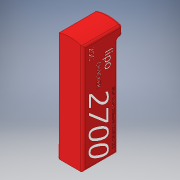
# Autodesk Inventor part: Akku_3S_2700
Saved by Autodesk Inventor 2017 SP1 (Build 210196100, 196)
## iProperties
Part Number: Akku_3S_2700
Material: Generisch
Document SubType Name: Modeling
Designer: Alex
Density: 1 g/cm^3
Appearance: Vorgabe
Author: Alex
Autodesk Inventor part; units mm, degrees
(part 1 of 2)
ref_plane "YZ Plane" through (0, 0, 0) normal (1, 0, 0) x (0, 1, 0)
ref_plane "XZ Plane" through (0, 0, 0) normal (0, 1, 0) x (-1, 0, 0)
ref_plane "XY Plane" through (0, 0, 0) normal (0, 0, 1) x (1, 0, 0)
sketch "Skizze1" plane through (0, 0, 0) normal (0, 1, 0) x (-1, 0, 0)
  line L0 (0, 0) -> (0, -110)
  line L1 (13, 23) -> (13, -138)
  arc A0 (13, 2.5038) -> (0, 0) centre (13, -32.4962) ccw
  line L2 (0, -110) -> (13, -110)
  line L3 (26, 0) -> (26, -110)
  arc A1 (26, 0) -> (13, 2.5038) centre (13, -32.4962) ccw
  line L4 (26, -110) -> (13, -110)
  dimension "d0" = 110
  dimension "d1" = 26
  dimension "d3" = 35
  constraints: 10 end point, 4 point on circle, 2 centre point, 2 point on line, 2 symmetric about line, 2 vertical, 1 perpendicular, 1 other
  measures "d0" distance of L0.start L0.end
  measures "d1" diameter of L0 L1
  measures "d3" radius of A0
extrude "Extrusion1" add sketch "Skizze1" along normal blind 35
sketch "Skizze2" plane through (0, 35, 0) normal (0, 1, 0) x (1, 0, 0)
  arc A0 (-26, 0) -> (0, 0) centre (-13, 32.4962) ccw projected
  arc A1 (-19.9948, -0.0016) -> (0, 0) centre (-10, 33.541) ccw
  line L0 (0, 0) -> (0, 110) projected
  line L1 (-26, 0) -> (-26, 10)
  line L2 (-26, 10) -> (0, 10)
  line L3 (0, 0) -> (0, 10)
  dimension "d6" = 10
  dimension "d7" = 35
  dimension "d8" = 10
  constraints: 6 end point, 2 perpendicular, 2 point on circle, 1 centre point, 1 point on line
  measures "d6" distance from line of L0 A1.centre
  measures "d7" radius of A1
  measures "d8" distance of L1.start L1.end
extrude "Extrusion2" add sketch "Skizze2" along normal blind 5
fillet "Rundung1" radius 2.5 2 edges at (-13, 35, -10) (-13, 40, -10)
fillet "Rundung2" radius 2.5 17 edges at (0, 17.5, -110) (-26, 17.5, -110) (0, 20, 0) (-26, 20, 0) (-13, 40, 2.5038) (0, 39.2678, -9.2678) (0, 37.5, -10) (0, 35.7322, -10.7322) (0, 35, -61.2499) (0, 40, -3.7501) (-26, 37.5, -10) (-26, 35.7322, -10.7322) (-26, 39.2678, -9.2678) (-26, 40, -3.75) (-26, 35, -61.2499) (0, 0, -55) (-26, 0, -55)
sketch "Skizze3" plane through (0, 2.5, -1.739) normal (1, 0, 0) x (0, 0, -1)
  line L0 (47.7852, 29.5) -> (102.261, 29.5) construction
  line L1 (102.261, 29.5) -> (102.261, 25.7703) construction
  line L2 (102.261, 25.7703) -> (47.7852, 25.7703) construction
  line L3 (47.7852, 25.7703) -> (47.7852, 29.5) construction
  line L4 (108.261, -2.5) -> (108.261, 32.5) projected
  line L5 (40.7159, 23.7627) -> (102.0936, 23.7627) construction
  line L6 (102.0936, 23.7627) -> (102.0936, 2.9199) construction
  line L7 (102.0936, 2.9199) -> (40.7159, 2.9199) construction
  line L8 (40.7159, 2.9199) -> (40.7159, 23.7627) construction
  line L9 (108.261, 32.5) -> (10.761, 32.5) projected
  line L10 (2.2367, 27.745) -> (43.751, 27.745) construction
  line L11 (43.751, 27.745) -> (43.751, 1.913) construction
  line L12 (43.751, 1.913) -> (2.2367, 1.913) construction
  line L13 (2.2367, 1.913) -> (2.2367, 27.745) construction
  line L14 (14.308, 19.3885) -> (13.2967, 19.3885)
  line L15 (13.2967, 19.3885) -> (13.2967, 27.745)
  line L16 (13.2967, 27.745) -> (14.308, 27.745)
  line L17 (14.308, 27.745) -> (14.308, 19.3885)
  line L18 (16.8234, 19.3885) -> (15.8121, 19.3885)
  line L19 (15.8121, 19.3885) -> (15.8121, 25.3917)
  line L20 (15.8121, 25.3917) -> (16.8234, 25.3917)
  line L21 (16.8234, 25.3917) -> (16.8234, 19.3885)
  line L22 (16.8947, 26.3901) -> (15.7472, 26.3901)
  line L23 (15.7472, 26.3901) -> (15.7472, 27.4403)
  line L24 (15.7472, 27.4403) -> (16.8947, 27.4403)
  line L25 (16.8947, 27.4403) -> (16.8947, 26.3901)
  spline S0 degree 2 poles (23.3388, 22.5521) (23.3388, 21.0481) (21.9061, 19.2718) (20.8104, 19.2718) knots 0 0 0 1 2 2 2
  spline S1 degree 2 poles (20.8104, 19.2718) (20.3631, 19.2718) (19.6759, 19.4792) (19.3194, 19.6932) knots 0 0 0 1 2 2 2
  line L26 (19.3194, 19.6932) -> (19.3194, 17.1778)
  line L27 (19.3194, 17.1778) -> (18.308, 17.1778)
  line L28 (18.308, 17.1778) -> (18.308, 25.3917)
  line L29 (18.308, 25.3917) -> (19.3194, 25.3917)
  line L30 (19.3194, 25.3917) -> (19.3194, 24.7628)
  spline S2 degree 2 poles (19.3194, 24.7628) (19.6954, 25.1064) (20.6159, 25.5603) (21.154, 25.5603) knots 0 0 0 1 2 2 2
  spline S3 degree 2 poles (21.154, 25.5603) (22.1848, 25.5603) (23.3388, 23.9265) (23.3388, 22.5521) knots 0 0 0 1 2 2 2
  spline S4 degree 2 poles (22.295, 22.4355) (22.295, 23.4662) (21.6403, 24.6008) (20.9077, 24.6008) knots 0 0 0 1 2 2 2
  spline S5 degree 2 poles (20.9077, 24.6008) (20.4798, 24.6008) (19.6759, 24.2183) (19.3194, 23.9201) knots 0 0 0 1 2 2 2
  line L31 (19.3194, 23.9201) -> (19.3194, 20.51)
  spline S6 degree 2 poles (19.3194, 20.51) (19.7148, 20.322) (20.2788, 20.1794) (20.6419, 20.1794) knots 0 0 0 1 2 2 2
  spline S7 degree 2 poles (20.6419, 20.1794) (21.4263, 20.1794) (22.295, 21.3333) (22.295, 22.4355) knots 0 0 0 1 2 2 2
  spline S8 degree 2 poles (29.3226, 22.3901) (29.3226, 20.8731) (27.8639, 19.2199) (26.6451, 19.2199) knots 0 0 0 1 2 2 2
  spline S9 degree 2 poles (26.6451, 19.2199) (25.3939, 19.2199) (23.9612, 20.9249) (23.9612, 22.3901) knots 0 0 0 1 2 2 2
  spline S10 degree 2 poles (23.9612, 22.3901) (23.9612, 23.8941) (25.4393, 25.5603) (26.6451, 25.5603) knots 0 0 0 1 2 2 2
  spline S11 degree 2 poles (26.6451, 25.5603) (27.8639, 25.5603) (29.3226, 23.9006) (29.3226, 22.3901) knots 0 0 0 1 2 2 2
  spline S12 degree 2 poles (28.2788, 22.3901) (28.2788, 23.557) (27.4296, 24.6915) (26.6451, 24.6915) knots 0 0 0 1 2 2 2
  spline S13 degree 2 poles (26.6451, 24.6915) (25.8607, 24.6915) (25.0049, 23.557) (25.0049, 22.3901) knots 0 0 0 1 2 2 2
  spline S14 degree 2 poles (25.0049, 22.3901) (25.0049, 21.2556) (25.8607, 20.0886) (26.6451, 20.0886) knots 0 0 0 1 2 2 2
  spline S15 degree 2 poles (26.6451, 20.0886) (27.4231, 20.0886) (28.2788, 21.2361) (28.2788, 22.3901) knots 0 0 0 1 2 2 2
  spline S16 degree 2 poles (20.7399, 11.1877) (20.351, 11.1877) (19.6929, 11.4502) (19.4531, 11.7128) knots 0 0 0 1 2 2 2
  spline S17 degree 2 poles (19.4531, 11.7128) (19.2132, 11.9721) (18.9506, 12.7501) (18.9506, 13.2557) knots 0 0 0 1 2 2 2
  spline S18 degree 2 poles (18.9506, 13.2557) (18.9506, 13.7582) (19.2067, 14.5037) (19.4498, 14.7792) knots 0 0 0 1 2 2 2
  spline S19 degree 2 poles (19.4498, 14.7792) (19.6897, 15.0483) (20.3445, 15.3303) (20.7497, 15.3303) knots 0 0 0 1 2 2 2
  spline S20 degree 2 poles (20.7497, 15.3303) (20.9506, 15.3303) (21.304, 15.2719) (21.4531, 15.2266) knots 0 0 0 1 2 2 2
  spline S21 degree 2 poles (21.4531, 15.2266) (21.5827, 15.1844) (21.8518, 15.0645) (21.9847, 14.9932) knots 0 0 0 1 2 2 2
  line L32 (21.9847, 14.9932) -> (21.9847, 14.3514)
  line L33 (21.9847, 14.3514) -> (21.9425, 14.3514)
  spline S22 degree 2 poles (21.9425, 14.3514) (21.8712, 14.4162) (21.6508, 14.5977) (21.492, 14.6852) knots 0 0 0 1 2 2 2
  spline S23 degree 2 poles (21.492, 14.6852) (21.3396, 14.7695) (20.9798, 14.8765) (20.7464, 14.8765) knots 0 0 0 1 2 2 2
  spline S24 degree 2 poles (20.7464, 14.8765) (20.4903, 14.8765) (20.0333, 14.6658) (19.8615, 14.4648) knots 0 0 0 1 2 2 2
  spline S25 degree 2 poles (19.8615, 14.4648) (19.6929, 14.2606) (19.5049, 13.6415) (19.5049, 13.2557) knots 0 0 0 1 2 2 2
  spline S26 degree 2 poles (19.5049, 13.2557) (19.5049, 12.8441) (19.7027, 12.2509) (19.8745, 12.0467) knots 0 0 0 1 2 2 2
  spline S27 degree 2 poles (19.8745, 12.0467) (20.043, 11.8489) (20.4936, 11.648) (20.7464, 11.648) knots 0 0 0 1 2 2 2
  spline S28 degree 2 poles (20.7464, 11.648) (20.9766, 11.648) (21.3688, 11.7614) (21.5211, 11.8457) knots 0 0 0 1 2 2 2
  spline S29 degree 2 poles (21.5211, 11.8457) (21.667, 11.93) (21.8842, 12.105) (21.9458, 12.1666) knots 0 0 0 1 2 2 2
  line L34 (21.9458, 12.1666) -> (21.9847, 12.1666)
  line L35 (21.9847, 12.1666) -> (21.9847, 11.5313)
  spline S30 degree 2 poles (21.9847, 11.5313) (21.8518, 11.4697) (21.6184, 11.3562) (21.4531, 11.3044) knots 0 0 0 1 2 2 2
  spline S31 degree 2 poles (21.4531, 11.3044) (21.278, 11.246) (20.9798, 11.1877) (20.7399, 11.1877) knots 0 0 0 1 2 2 2
  line L36 (25.5762, 11.259) -> (24.8858, 11.259)
  line L37 (24.8858, 11.259) -> (23.6216, 12.8506)
  line L38 (23.6216, 12.8506) -> (23.0122, 12.8506)
  line L39 (23.0122, 12.8506) -> (23.0122, 11.259)
  line L40 (23.0122, 11.259) -> (22.4806, 11.259)
  line L41 (22.4806, 11.259) -> (22.4806, 15.259)
  line L42 (22.4806, 15.259) -> (23.5114, 15.259)
  spline S32 degree 2 poles (23.5114, 15.259) (23.855, 15.259) (24.3185, 15.1844) (24.5292, 15.0483) knots 0 0 0 1 2 2 2
  spline S33 degree 2 poles (24.5292, 15.0483) (24.7399, 14.9121) (24.983, 14.4875) (24.983, 14.1731) knots 0 0 0 1 2 2 2
  spline S34 degree 2 poles (24.983, 14.1731) (24.983, 13.7355) (24.5357, 13.1423) (24.1532, 12.9997) knots 0 0 0 1 2 2 2
  line L43 (24.1532, 12.9997) -> (25.5762, 11.259)
  spline S35 degree 2 poles (24.4288, 14.1309) (24.4288, 14.306) (24.3056, 14.575) (24.1759, 14.6625) knots 0 0 0 1 2 2 2
  spline S36 degree 2 poles (24.1759, 14.6625) (24.0625, 14.7371) (23.761, 14.7987) (23.5406, 14.7987) knots 0 0 0 1 2 2 2
  line L44 (23.5406, 14.7987) -> (23.0122, 14.7987)
  line L45 (23.0122, 14.7987) -> (23.0122, 13.2946)
  line L46 (23.0122, 13.2946) -> (23.479, 13.2946)
  spline S37 degree 2 poles (23.479, 13.2946) (23.7091, 13.2946) (24.0754, 13.3757) (24.2018, 13.5021) knots 0 0 0 1 2 2 2
  spline S38 degree 2 poles (24.2018, 13.5021) (24.3185, 13.6123) (24.4288, 13.9235) (24.4288, 14.1309) knots 0 0 0 1 2 2 2
  line L47 (25.4628, 11.259) -> (26.8112, 15.259)
  line L48 (26.8112, 15.259) -> (27.466, 15.259)
  line L49 (27.466, 15.259) -> (28.8145, 11.259)
  line L50 (28.8145, 11.259) -> (28.2537, 11.259)
  line L51 (28.2537, 11.259) -> (27.8907, 12.3773)
  line L52 (27.8907, 12.3773) -> (26.3639, 12.3773)
  line L53 (26.3639, 12.3773) -> (26.0009, 11.259)
  line L54 (26.0009, 11.259) -> (25.4628, 11.259)
  line L55 (27.7448, 12.8311) -> (27.1257, 14.7144)
  line L56 (27.1257, 14.7144) -> (26.5098, 12.8311)
  line L57 (26.5098, 12.8311) -> (27.7448, 12.8311)
  spline S39 degree 2 poles (30.7561, 11.1877) (30.3672, 11.1877) (29.7091, 11.4502) (29.4693, 11.7128) knots 0 0 0 1 2 2 2
  spline S40 degree 2 poles (29.4693, 11.7128) (29.2294, 11.9721) (28.9668, 12.7501) (28.9668, 13.2557) knots 0 0 0 1 2 2 2
  spline S41 degree 2 poles (28.9668, 13.2557) (28.9668, 13.7582) (29.2229, 14.5037) (29.466, 14.7792) knots 0 0 0 1 2 2 2
  spline S42 degree 2 poles (29.466, 14.7792) (29.7059, 15.0483) (30.3607, 15.3303) (30.7659, 15.3303) knots 0 0 0 1 2 2 2
  spline S43 degree 2 poles (30.7659, 15.3303) (30.9668, 15.3303) (31.3202, 15.2719) (31.4693, 15.2266) knots 0 0 0 1 2 2 2
  spline S44 degree 2 poles (31.4693, 15.2266) (31.5989, 15.1844) (31.868, 15.0645) (32.0009, 14.9932) knots 0 0 0 1 2 2 2
  line L58 (32.0009, 14.9932) -> (32.0009, 14.3514)
  line L59 (32.0009, 14.3514) -> (31.9587, 14.3514)
  spline S45 degree 2 poles (31.9587, 14.3514) (31.8874, 14.4162) (31.667, 14.5977) (31.5082, 14.6852) knots 0 0 0 1 2 2 2
  spline S46 degree 2 poles (31.5082, 14.6852) (31.3558, 14.7695) (30.996, 14.8765) (30.7626, 14.8765) knots 0 0 0 1 2 2 2
  spline S47 degree 2 poles (30.7626, 14.8765) (30.5065, 14.8765) (30.0495, 14.6658) (29.8777, 14.4648) knots 0 0 0 1 2 2 2
  spline S48 degree 2 poles (29.8777, 14.4648) (29.7091, 14.2606) (29.5211, 13.6415) (29.5211, 13.2557) knots 0 0 0 1 2 2 2
  spline S49 degree 2 poles (29.5211, 13.2557) (29.5211, 12.8441) (29.7189, 12.2509) (29.8907, 12.0467) knots 0 0 0 1 2 2 2
  spline S50 degree 2 poles (29.8907, 12.0467) (30.0592, 11.8489) (30.5098, 11.648) (30.7626, 11.648) knots 0 0 0 1 2 2 2
  spline S51 degree 2 poles (30.7626, 11.648) (30.9928, 11.648) (31.385, 11.7614) (31.5373, 11.8457) knots 0 0 0 1 2 2 2
  spline S52 degree 2 poles (31.5373, 11.8457) (31.6832, 11.93) (31.9004, 12.105) (31.962, 12.1666) knots 0 0 0 1 2 2 2
  line L60 (31.962, 12.1666) -> (32.0009, 12.1666)
  line L61 (32.0009, 12.1666) -> (32.0009, 11.5313)
  spline S53 degree 2 poles (32.0009, 11.5313) (31.868, 11.4697) (31.6346, 11.3562) (31.4693, 11.3044) knots 0 0 0 1 2 2 2
  spline S54 degree 2 poles (31.4693, 11.3044) (31.2942, 11.246) (30.996, 11.1877) (30.7561, 11.1877) knots 0 0 0 1 2 2 2
  line L62 (35.4142, 11.259) -> (34.7237, 11.259)
  line L63 (34.7237, 11.259) -> (33.2618, 13.1196)
  line L64 (33.2618, 13.1196) -> (33.0284, 12.857)
  line L65 (33.0284, 12.857) -> (33.0284, 11.259)
  line L66 (33.0284, 11.259) -> (32.4968, 11.259)
  line L67 (32.4968, 11.259) -> (32.4968, 15.259)
  line L68 (32.4968, 15.259) -> (33.0284, 15.259)
  line L69 (33.0284, 15.259) -> (33.0284, 13.4211)
  line L70 (33.0284, 13.4211) -> (34.6686, 15.259)
  line L71 (34.6686, 15.259) -> (35.3169, 15.259)
  line L72 (35.3169, 15.259) -> (33.6605, 13.4729)
  line L73 (33.6605, 13.4729) -> (35.4142, 11.259)
  line L74 (35.7318, 11.259) -> (35.7318, 15.259)
  line L75 (35.7318, 15.259) -> (38.2343, 15.259)
  line L76 (38.2343, 15.259) -> (38.2343, 14.7857)
  line L77 (38.2343, 14.7857) -> (36.2634, 14.7857)
  line L78 (36.2634, 14.7857) -> (36.2634, 13.6901)
  line L79 (36.2634, 13.6901) -> (38.1014, 13.6901)
  line L80 (38.1014, 13.6901) -> (38.1014, 13.2168)
  line L81 (38.1014, 13.2168) -> (36.2634, 13.2168)
  line L82 (36.2634, 13.2168) -> (36.2634, 11.7322)
  line L83 (36.2634, 11.7322) -> (38.2343, 11.7322)
  line L84 (38.2343, 11.7322) -> (38.2343, 11.259)
  line L85 (38.2343, 11.259) -> (35.7318, 11.259)
  line L86 (41.9134, 11.259) -> (41.2229, 11.259)
  line L87 (41.2229, 11.259) -> (39.9587, 12.8506)
  line L88 (39.9587, 12.8506) -> (39.3493, 12.8506)
  line L89 (39.3493, 12.8506) -> (39.3493, 11.259)
  line L90 (39.3493, 11.259) -> (38.8177, 11.259)
  line L91 (38.8177, 11.259) -> (38.8177, 15.259)
  line L92 (38.8177, 15.259) -> (39.8485, 15.259)
  spline S55 degree 2 poles (39.8485, 15.259) (40.1921, 15.259) (40.6557, 15.1844) (40.8664, 15.0483) knots 0 0 0 1 2 2 2
  spline S56 degree 2 poles (40.8664, 15.0483) (41.0771, 14.9121) (41.3202, 14.4875) (41.3202, 14.1731) knots 0 0 0 1 2 2 2
  spline S57 degree 2 poles (41.3202, 14.1731) (41.3202, 13.7355) (40.8728, 13.1423) (40.4903, 12.9997) knots 0 0 0 1 2 2 2
  line L93 (40.4903, 12.9997) -> (41.9134, 11.259)
  spline S58 degree 2 poles (40.7659, 14.1309) (40.7659, 14.306) (40.6427, 14.575) (40.513, 14.6625) knots 0 0 0 1 2 2 2
  spline S59 degree 2 poles (40.513, 14.6625) (40.3996, 14.7371) (40.0981, 14.7987) (39.8777, 14.7987) knots 0 0 0 1 2 2 2
  line L94 (39.8777, 14.7987) -> (39.3493, 14.7987)
  line L95 (39.3493, 14.7987) -> (39.3493, 13.2946)
  line L96 (39.3493, 13.2946) -> (39.8161, 13.2946)
  spline S60 degree 2 poles (39.8161, 13.2946) (40.0463, 13.2946) (40.4125, 13.3757) (40.539, 13.5021) knots 0 0 0 1 2 2 2
  spline S61 degree 2 poles (40.539, 13.5021) (40.6557, 13.6123) (40.7659, 13.9235) (40.7659, 14.1309) knots 0 0 0 1 2 2 2
  line L97 (5.6848, 3.4125) -> (2.6014, 3.4125)
  line L98 (2.6014, 3.4125) -> (2.6014, 4.1216)
  spline S62 degree 2 poles (2.6014, 4.1216) (2.9336, 4.4336) (3.5252, 5.013) (3.8088, 5.325) knots 0 0 0 1 2 2 2
  spline S63 degree 2 poles (3.8088, 5.325) (4.3801, 5.953) (4.7975, 6.7067) (4.7975, 7.1078) knots 0 0 0 1 2 2 2
  spline S64 degree 2 poles (4.7975, 7.1078) (4.7975, 7.3185) (4.6678, 7.6345) (4.5503, 7.7358) knots 0 0 0 1 2 2 2
  spline S65 degree 2 poles (4.5503, 7.7358) (4.4328, 7.8371) (4.1249, 7.9384) (3.9385, 7.9384) knots 0 0 0 1 2 2 2
  spline S66 degree 2 poles (3.9385, 7.9384) (3.7602, 7.9384) (3.3955, 7.8493) (3.2294, 7.7804) knots 0 0 0 1 2 2 2
  spline S67 degree 2 poles (3.2294, 7.7804) (3.0876, 7.7237) (2.8242, 7.5616) (2.7432, 7.5049) knots 0 0 0 1 2 2 2
  line L99 (2.7432, 7.5049) -> (2.7067, 7.5049)
  line L100 (2.7067, 7.5049) -> (2.7067, 8.218)
  spline S68 degree 2 poles (2.7067, 8.218) (2.9134, 8.3193) (3.6548, 8.5179) (3.9871, 8.5179) knots 0 0 0 1 2 2 2
  spline S69 degree 2 poles (3.9871, 8.5179) (4.6881, 8.5179) (5.4782, 7.7764) (5.4782, 7.1443) knots 0 0 0 1 2 2 2
  spline S70 degree 2 poles (5.4782, 7.1443) (5.4782, 6.8485) (5.3404, 6.3542) (5.2189, 6.1435) knots 0 0 0 1 2 2 2
  spline S71 degree 2 poles (5.2189, 6.1435) (5.0973, 5.9247) (4.7448, 5.4952) (4.5503, 5.2885) knots 0 0 0 1 2 2 2
  spline S72 degree 2 poles (4.5503, 5.2885) (4.2343, 4.9441) (3.4604, 4.2067) (3.2294, 3.9919) knots 0 0 0 1 2 2 2
  line L101 (3.2294, 3.9919) -> (5.6848, 3.9919)
  line L102 (5.6848, 3.9919) -> (5.6848, 3.4125)
  spline S73 degree 2 poles (9.3842, 5.0008) (9.3842, 4.6402) (9.1532, 4.0243) (8.9425, 3.7974) knots 0 0 0 1 2 2 2
  spline S74 degree 2 poles (8.9425, 3.7974) (8.7318, 3.5705) (8.1038, 3.3072) (7.7148, 3.3072) knots 0 0 0 1 2 2 2
  spline S75 degree 2 poles (7.7148, 3.3072) (7.3582, 3.3072) (6.6613, 3.4652) (6.4061, 3.5908) knots 0 0 0 1 2 2 2
  line L103 (6.4061, 3.5908) -> (6.4061, 4.2999)
  line L104 (6.4061, 4.2999) -> (6.4547, 4.2999)
  spline S76 degree 2 poles (6.4547, 4.2999) (6.5317, 4.2431) (6.8194, 4.0973) (6.9936, 4.0324) knots 0 0 0 1 2 2 2
  spline S77 degree 2 poles (6.9936, 4.0324) (7.1921, 3.9636) (7.5203, 3.8866) (7.727, 3.8866) knots 0 0 0 1 2 2 2
  spline S78 degree 2 poles (7.727, 3.8866) (7.9296, 3.8866) (8.3104, 4.0324) (8.4482, 4.1905) knots 0 0 0 1 2 2 2
  spline S79 degree 2 poles (8.4482, 4.1905) (8.5738, 4.3404) (8.7035, 4.7375) (8.7035, 5.0049) knots 0 0 0 1 2 2 2
  spline S80 degree 2 poles (8.7035, 5.0049) (8.7035, 5.2723) (8.5576, 5.6127) (8.4198, 5.7261) knots 0 0 0 1 2 2 2
  spline S81 degree 2 poles (8.4198, 5.7261) (8.278, 5.8517) (7.8566, 5.9571) (7.6014, 5.9571) knots 0 0 0 1 2 2 2
  spline S82 degree 2 poles (7.6014, 5.9571) (7.3258, 5.9571) (6.7788, 5.872) (6.6127, 5.8355) knots 0 0 0 1 2 2 2
  line L105 (6.6127, 5.8355) -> (6.6127, 8.4125)
  line L106 (6.6127, 8.4125) -> (9.3558, 8.4125)
  line L107 (9.3558, 8.4125) -> (9.3558, 7.825)
  line L108 (9.3558, 7.825) -> (7.257, 7.825)
  line L109 (7.257, 7.825) -> (7.257, 6.4919)
  spline S83 degree 2 poles (7.257, 6.4919) (7.3785, 6.5081) (7.6135, 6.5203) (7.7108, 6.5203) knots 0 0 0 1 2 2 2
  spline S84 degree 2 poles (7.7108, 6.5203) (8.0957, 6.5203) (8.6265, 6.3947) (8.8696, 6.2083) knots 0 0 0 1 2 2 2
  spline S85 degree 2 poles (8.8696, 6.2083) (9.1168, 6.0219) (9.3842, 5.4546) (9.3842, 5.0008) knots 0 0 0 1 2 2 2
  spline S86 degree 2 poles (12.2002, 3.3234) (11.714, 3.3234) (10.8915, 3.6516) (10.5916, 3.9798) knots 0 0 0 1 2 2 2
  spline S87 degree 2 poles (10.5916, 3.9798) (10.2918, 4.3039) (9.9636, 5.2764) (9.9636, 5.9085) knots 0 0 0 1 2 2 2
  spline S88 degree 2 poles (9.9636, 5.9085) (9.9636, 6.5365) (10.2837, 7.4684) (10.5876, 7.8128) knots 0 0 0 1 2 2 2
  spline S89 degree 2 poles (10.5876, 7.8128) (10.8874, 8.1491) (11.7059, 8.5016) (12.2124, 8.5016) knots 0 0 0 1 2 2 2
  spline S90 degree 2 poles (12.2124, 8.5016) (12.4636, 8.5016) (12.9053, 8.4287) (13.0916, 8.372) knots 0 0 0 1 2 2 2
  spline S91 degree 2 poles (13.0916, 8.372) (13.2537, 8.3193) (13.59, 8.1694) (13.7561, 8.0803) knots 0 0 0 1 2 2 2
  line L110 (13.7561, 8.0803) -> (13.7561, 7.278)
  line L111 (13.7561, 7.278) -> (13.7035, 7.278)
  spline S92 degree 2 poles (13.7035, 7.278) (13.6143, 7.359) (13.3388, 7.5859) (13.1403, 7.6953) knots 0 0 0 1 2 2 2
  spline S93 degree 2 poles (13.1403, 7.6953) (12.9498, 7.8007) (12.5001, 7.9344) (12.2083, 7.9344) knots 0 0 0 1 2 2 2
  spline S94 degree 2 poles (12.2083, 7.9344) (11.8882, 7.9344) (11.3169, 7.671) (11.1022, 7.4198) knots 0 0 0 1 2 2 2
  spline S95 degree 2 poles (11.1022, 7.4198) (10.8915, 7.1645) (10.6565, 6.3906) (10.6565, 5.9085) knots 0 0 0 1 2 2 2
  spline S96 degree 2 poles (10.6565, 5.9085) (10.6565, 5.3939) (10.9036, 4.6524) (11.1184, 4.3971) knots 0 0 0 1 2 2 2
  spline S97 degree 2 poles (11.1184, 4.3971) (11.3291, 4.1499) (11.8923, 3.8987) (12.2083, 3.8987) knots 0 0 0 1 2 2 2
  spline S98 degree 2 poles (12.2083, 3.8987) (12.496, 3.8987) (12.9863, 4.0405) (13.1767, 4.1459) knots 0 0 0 1 2 2 2
  spline S99 degree 2 poles (13.1767, 4.1459) (13.3591, 4.2512) (13.6305, 4.47) (13.7075, 4.547) knots 0 0 0 1 2 2 2
  line L112 (13.7075, 4.547) -> (13.7561, 4.547)
  line L113 (13.7561, 4.547) -> (13.7561, 3.7529)
  spline S100 degree 2 poles (13.7561, 3.7529) (13.59, 3.6759) (13.2983, 3.5341) (13.0916, 3.4692) knots 0 0 0 1 2 2 2
  spline S101 degree 2 poles (13.0916, 3.4692) (12.8728, 3.3963) (12.5001, 3.3234) (12.2002, 3.3234) knots 0 0 0 1 2 2 2
  line L114 (54.5085, 3.3413) -> (42.1746, 3.3413)
  line L115 (42.1746, 3.3413) -> (43.1308, 6.1776)
  spline S102 degree 2 poles (43.1308, 6.1776) (44.8975, 7.4256) (48.0417, 9.7432) (49.5976, 10.9912) knots 0 0 0 1 2 2 2
  spline S103 degree 2 poles (49.5976, 10.9912) (52.7419, 13.5034) (55.4323, 16.5179) (55.9833, 18.1225) knots 0 0 0 1 2 2 2
  spline S104 degree 2 poles (55.9833, 18.1225) (56.2751, 18.9653) (56.1778, 20.2295) (55.8537, 20.6346) knots 0 0 0 1 2 2 2
  spline S105 degree 2 poles (55.8537, 20.6346) (55.5295, 21.0398) (54.4274, 21.445) (53.6819, 21.445) knots 0 0 0 1 2 2 2
  spline S106 degree 2 poles (53.6819, 21.445) (52.9688, 21.445) (51.3804, 21.0884) (50.6187, 20.8129) knots 0 0 0 1 2 2 2
  spline S107 degree 2 poles (50.6187, 20.8129) (49.9704, 20.586) (48.7062, 19.9377) (48.301, 19.7108) knots 0 0 0 1 2 2 2
  line L116 (48.301, 19.7108) -> (48.1551, 19.7108)
  line L117 (48.1551, 19.7108) -> (49.1276, 22.5633)
  spline S108 degree 2 poles (49.1276, 22.5633) (50.1, 22.9685) (53.3415, 23.7627) (54.6705, 23.7627) knots 0 0 0 1 2 2 2
  spline S109 degree 2 poles (54.6705, 23.7627) (57.4582, 23.7627) (59.6138, 20.7967) (58.7548, 18.2684) knots 0 0 0 1 2 2 2
  spline S110 degree 2 poles (58.7548, 18.2684) (58.3496, 17.0852) (57.1341, 15.1079) (56.3561, 14.2651) knots 0 0 0 1 2 2 2
  spline S111 degree 2 poles (56.3561, 14.2651) (55.562, 13.3899) (53.5846, 11.6719) (52.5312, 10.8453) knots 0 0 0 1 2 2 2
  spline S112 degree 2 poles (52.5312, 10.8453) (50.797, 9.4677) (46.6965, 6.5179) (45.4809, 5.659) knots 0 0 0 1 2 2 2
  line L118 (45.4809, 5.659) -> (55.3026, 5.659)
  line L119 (55.3026, 5.659) -> (54.5085, 3.3413)
  line L120 (75.5295, 20.3429) -> (61.0887, 3.3413)
  line L121 (61.0887, 3.3413) -> (58.2362, 3.3413)
  line L122 (58.2362, 3.3413) -> (73.3739, 20.9912)
  line L123 (73.3739, 20.9912) -> (63.0498, 20.9912)
  line L124 (63.0498, 20.9912) -> (63.844, 23.3413)
  line L125 (63.844, 23.3413) -> (76.5344, 23.3413)
  line L126 (76.5344, 23.3413) -> (75.5295, 20.3429)
  spline S113 degree 2 poles (88.0417, 13.3413) (86.2103, 7.9604) (81.3642, 2.9199) (78.1065, 2.9199) knots 0 0 0 1 2 2 2
  spline S114 degree 2 poles (78.1065, 2.9199) (74.8002, 2.9199) (73.455, 8.0577) (75.2378, 13.3251) knots 0 0 0 1 2 2 2
  spline S115 degree 2 poles (75.2378, 13.3251) (77.0855, 18.7384) (81.9153, 23.7465) (85.173, 23.7465) knots 0 0 0 1 2 2 2
  spline S116 degree 2 poles (85.173, 23.7465) (88.4793, 23.7465) (89.8083, 18.5601) (88.0417, 13.3413) knots 0 0 0 1 2 2 2
  spline S117 degree 2 poles (82.5312, 7.2473) (83.2605, 8.2359) (84.6057, 11.2829) (85.3188, 13.3413) knots 0 0 0 1 2 2 2
  spline S118 degree 2 poles (85.3188, 13.3413) (86.0158, 15.3996) (86.7289, 18.4304) (86.6641, 19.4515) knots 0 0 0 1 2 2 2
  spline S119 degree 2 poles (86.6641, 19.4515) (86.5992, 20.4726) (85.562, 21.526) (84.4274, 21.526) knots 0 0 0 1 2 2 2
  spline S120 degree 2 poles (84.4274, 21.526) (83.3091, 21.526) (81.5101, 20.4726) (80.7321, 19.4191) knots 0 0 0 1 2 2 2
  spline S121 degree 2 poles (80.7321, 19.4191) (79.9866, 18.398) (78.6252, 15.2862) (77.9607, 13.3251) knots 0 0 0 1 2 2 2
  spline S122 degree 2 poles (77.9607, 13.3251) (77.2475, 11.2181) (76.5506, 8.398) (76.5992, 7.2959) knots 0 0 0 1 2 2 2
  spline S123 degree 2 poles (76.5992, 7.2959) (76.6316, 6.2586) (77.7013, 5.1403) (78.8521, 5.1403) knots 0 0 0 1 2 2 2
  spline S124 degree 2 poles (78.8521, 5.1403) (79.9704, 5.1403) (81.7694, 6.1938) (82.5312, 7.2473) knots 0 0 0 1 2 2 2
  spline S125 degree 2 poles (103.0498, 13.3413) (101.2184, 7.9604) (96.3723, 2.9199) (93.1146, 2.9199) knots 0 0 0 1 2 2 2
  spline S126 degree 2 poles (93.1146, 2.9199) (89.8083, 2.9199) (88.4631, 8.0577) (90.2459, 13.3251) knots 0 0 0 1 2 2 2
  spline S127 degree 2 poles (90.2459, 13.3251) (92.0936, 18.7384) (96.9234, 23.7465) (100.1811, 23.7465) knots 0 0 0 1 2 2 2
  spline S128 degree 2 poles (100.1811, 23.7465) (103.4874, 23.7465) (104.8164, 18.5601) (103.0498, 13.3413) knots 0 0 0 1 2 2 2
  spline S129 degree 2 poles (97.5393, 7.2473) (98.2686, 8.2359) (99.6138, 11.2829) (100.3269, 13.3413) knots 0 0 0 1 2 2 2
  spline S130 degree 2 poles (100.3269, 13.3413) (101.0239, 15.3996) (101.737, 18.4304) (101.6722, 19.4515) knots 0 0 0 1 2 2 2
  spline S131 degree 2 poles (101.6722, 19.4515) (101.6073, 20.4726) (100.5701, 21.526) (99.4355, 21.526) knots 0 0 0 1 2 2 2
  spline S132 degree 2 poles (99.4355, 21.526) (98.3172, 21.526) (96.5182, 20.4726) (95.7402, 19.4191) knots 0 0 0 1 2 2 2
  spline S133 degree 2 poles (95.7402, 19.4191) (94.9947, 18.398) (93.6333, 15.2862) (92.9688, 13.3251) knots 0 0 0 1 2 2 2
  spline S134 degree 2 poles (92.9688, 13.3251) (92.2556, 11.2181) (91.5587, 8.398) (91.6073, 7.2959) knots 0 0 0 1 2 2 2
  spline S135 degree 2 poles (91.6073, 7.2959) (91.6398, 6.2586) (92.7094, 5.1403) (93.8602, 5.1403) knots 0 0 0 1 2 2 2
  spline S136 degree 2 poles (93.8602, 5.1403) (94.9785, 5.1403) (96.7775, 6.1938) (97.5393, 7.2473) knots 0 0 0 1 2 2 2
  spline S137 degree 2 poles (48.6422, 29.1515) (48.551, 29.1515) (48.3707, 29.107) (48.2836, 29.0725) knots 0 0 0 1 2 2 2
  spline S138 degree 2 poles (48.2836, 29.0725) (48.2025, 29.0381) (48.083, 28.9652) (48.0364, 28.9327) knots 0 0 0 1 2 2 2
  line L127 (48.0364, 28.9327) -> (48.0161, 28.9327)
  line L128 (48.0161, 28.9327) -> (48.0161, 29.2873)
  spline S139 degree 2 poles (48.0161, 29.2873) (48.1255, 29.346) (48.5003, 29.4412) (48.6685, 29.4412) knots 0 0 0 1 2 2 2
  spline S140 degree 2 poles (48.6685, 29.4412) (48.8387, 29.4412) (49.0919, 29.3724) (49.1952, 29.2994) knots 0 0 0 1 2 2 2
  spline S141 degree 2 poles (49.1952, 29.2994) (49.3046, 29.2204) (49.4181, 28.9915) (49.4181, 28.8375) knots 0 0 0 1 2 2 2
  spline S142 degree 2 poles (49.4181, 28.8375) (49.4181, 28.6309) (49.1466, 28.3189) (48.9562, 28.2784) knots 0 0 0 1 2 2 2
  line L129 (48.9562, 28.2784) -> (48.9562, 28.2541)
  spline S143 degree 2 poles (48.9562, 28.2541) (49.0352, 28.2378) (49.2155, 28.1649) (49.2925, 28.092) knots 0 0 0 1 2 2 2
  spline S144 degree 2 poles (49.2925, 28.092) (49.3695, 28.0211) (49.4667, 27.7942) (49.4667, 27.6301) knots 0 0 0 1 2 2 2
  spline S145 degree 2 poles (49.4667, 27.6301) (49.4667, 27.4619) (49.3512, 27.1763) (49.2459, 27.0669) knots 0 0 0 1 2 2 2
  spline S146 degree 2 poles (49.2459, 27.0669) (49.1365, 26.9534) (48.8265, 26.8359) (48.63, 26.8359) knots 0 0 0 1 2 2 2
  spline S147 degree 2 poles (48.63, 26.8359) (48.4416, 26.8359) (48.0729, 26.9271) (47.9473, 26.9899) knots 0 0 0 1 2 2 2
  line L130 (47.9473, 26.9899) -> (47.9473, 27.3444)
  line L131 (47.9473, 27.3444) -> (47.9716, 27.3444)
  spline S148 degree 2 poles (47.9716, 27.3444) (48.0769, 27.2674) (48.4335, 27.1256) (48.6097, 27.1256) knots 0 0 0 1 2 2 2
  spline S149 degree 2 poles (48.6097, 27.1256) (48.7131, 27.1256) (48.9197, 27.1904) (48.9886, 27.2654) knots 0 0 0 1 2 2 2
  spline S150 degree 2 poles (48.9886, 27.2654) (49.0555, 27.3404) (49.1264, 27.5186) (49.1264, 27.6544) knots 0 0 0 1 2 2 2
  spline S151 degree 2 poles (49.1264, 27.6544) (49.1264, 27.7901) (49.0473, 27.9664) (48.9764, 28.017) knots 0 0 0 1 2 2 2
  spline S152 degree 2 poles (48.9764, 28.017) (48.9055, 28.0677) (48.7131, 28.1062) (48.5996, 28.1062) knots 0 0 0 1 2 2 2
  line L132 (48.5996, 28.1062) -> (48.4578, 28.1062)
  line L133 (48.4578, 28.1062) -> (48.4578, 28.3837)
  line L134 (48.4578, 28.3837) -> (48.5692, 28.3837)
  spline S153 degree 2 poles (48.5692, 28.3837) (48.7941, 28.3837) (49.0777, 28.5985) (49.0777, 28.8031) knots 0 0 0 1 2 2 2
  spline S154 degree 2 poles (49.0777, 28.8031) (49.0777, 28.8983) (49.0048, 29.034) (48.9461, 29.0746) knots 0 0 0 1 2 2 2
  spline S155 degree 2 poles (48.9461, 29.0746) (48.8832, 29.1171) (48.7293, 29.1515) (48.6422, 29.1515) knots 0 0 0 1 2 2 2
  spline S156 degree 2 poles (50.6114, 26.844) (50.3399, 26.844) (49.959, 26.9575) (49.7909, 27.0385) knots 0 0 0 1 2 2 2
  line L135 (49.7909, 27.0385) -> (49.7909, 27.4558)
  line L136 (49.7909, 27.4558) -> (49.8152, 27.4558)
  spline S157 degree 2 poles (49.8152, 27.4558) (49.9793, 27.3019) (50.3946, 27.1317) (50.5871, 27.1317) knots 0 0 0 1 2 2 2
  spline S158 degree 2 poles (50.5871, 27.1317) (50.8626, 27.1317) (51.1442, 27.3606) (51.1442, 27.549) knots 0 0 0 1 2 2 2
  spline S159 degree 2 poles (51.1442, 27.549) (51.1442, 27.6989) (50.9963, 27.8853) (50.8362, 27.9319) knots 0 0 0 1 2 2 2
  spline S160 degree 2 poles (50.8362, 27.9319) (50.7208, 27.9643) (50.5283, 28.0089) (50.3845, 28.0454) knots 0 0 0 1 2 2 2
  spline S161 degree 2 poles (50.3845, 28.0454) (50.2548, 28.0798) (50.0502, 28.1831) (49.9712, 28.2662) knots 0 0 0 1 2 2 2
  spline S162 degree 2 poles (49.9712, 28.2662) (49.8942, 28.3493) (49.8091, 28.5721) (49.8091, 28.718) knots 0 0 0 1 2 2 2
  spline S163 degree 2 poles (49.8091, 28.718) (49.8091, 29.0219) (50.2832, 29.4331) (50.6499, 29.4331) knots 0 0 0 1 2 2 2
  spline S164 degree 2 poles (50.6499, 29.4331) (50.8606, 29.4331) (51.2333, 29.3501) (51.3934, 29.2711) knots 0 0 0 1 2 2 2
  line L137 (51.3934, 29.2711) -> (51.3934, 28.874)
  line L138 (51.3934, 28.874) -> (51.3691, 28.874)
  spline S165 degree 2 poles (51.3691, 28.874) (51.2495, 28.9834) (50.8768, 29.1455) (50.6721, 29.1455) knots 0 0 0 1 2 2 2
  spline S166 degree 2 poles (50.6721, 29.1455) (50.4412, 29.1455) (50.1555, 28.9287) (50.1555, 28.7524) knots 0 0 0 1 2 2 2
  spline S167 degree 2 poles (50.1555, 28.7524) (50.1555, 28.5944) (50.3237, 28.406) (50.4817, 28.3635) knots 0 0 0 1 2 2 2
  spline S168 degree 2 poles (50.4817, 28.3635) (50.5871, 28.3351) (50.893, 28.2622) (50.9943, 28.2318) knots 0 0 0 1 2 2 2
  spline S169 degree 2 poles (50.9943, 28.2318) (51.2516, 28.1528) (51.4906, 27.8347) (51.4906, 27.6017) knots 0 0 0 1 2 2 2
  spline S170 degree 2 poles (51.4906, 27.6017) (51.4906, 27.4538) (51.3711, 27.1702) (51.2637, 27.0709) knots 0 0 0 1 2 2 2
  spline S171 degree 2 poles (51.2637, 27.0709) (51.1442, 26.9615) (50.8403, 26.844) (50.6114, 26.844) knots 0 0 0 1 2 2 2
  line L139 (53.1742, 26.8886) -> (51.9546, 26.8886)
  line L140 (51.9546, 26.8886) -> (51.9546, 27.1438)
  line L141 (51.9546, 27.1438) -> (52.4084, 27.1438)
  line L142 (52.4084, 27.1438) -> (52.4084, 28.8193)
  line L143 (52.4084, 28.8193) -> (51.9546, 28.8193)
  line L144 (51.9546, 28.8193) -> (51.9546, 29.0482)
  spline S172 degree 2 poles (51.9546, 29.0482) (52.2119, 29.0482) (52.455, 29.1941) (52.4712, 29.3967) knots 0 0 0 1 2 2 2
  line L145 (52.4712, 29.3967) -> (52.7305, 29.3967)
  line L146 (52.7305, 29.3967) -> (52.7305, 27.1438)
  line L147 (52.7305, 27.1438) -> (53.1742, 27.1438)
  line L148 (53.1742, 27.1438) -> (53.1742, 26.8886)
  spline S173 degree 2 poles (55.2852, 28.6349) (55.2852, 28.4729) (55.1697, 28.1811) (55.0664, 28.0798) knots 0 0 0 1 2 2 2
  spline S174 degree 2 poles (55.0664, 28.0798) (54.9367, 27.9522) (54.5862, 27.8205) (54.3188, 27.8205) knots 0 0 0 1 2 2 2
  line L149 (54.3188, 27.8205) -> (54.0372, 27.8205)
  line L150 (54.0372, 27.8205) -> (54.0372, 26.8886)
  line L151 (54.0372, 26.8886) -> (53.705, 26.8886)
  line L152 (53.705, 26.8886) -> (53.705, 29.3886)
  line L153 (53.705, 29.3886) -> (54.333, 29.3886)
  spline S175 degree 2 poles (54.333, 29.3886) (54.5559, 29.3886) (54.8679, 29.3156) (54.9874, 29.2326) knots 0 0 0 1 2 2 2
  spline S176 degree 2 poles (54.9874, 29.2326) (55.1272, 29.1374) (55.2852, 28.8436) (55.2852, 28.6349) knots 0 0 0 1 2 2 2
  spline S177 degree 2 poles (54.9388, 28.6248) (54.9388, 28.7545) (54.8496, 28.9449) (54.7584, 29.0057) knots 0 0 0 1 2 2 2
  spline S178 degree 2 poles (54.7584, 29.0057) (54.6794, 29.0583) (54.4687, 29.1009) (54.3127, 29.1009) knots 0 0 0 1 2 2 2
  line L154 (54.3127, 29.1009) -> (54.0372, 29.1009)
  line L155 (54.0372, 29.1009) -> (54.0372, 28.1041)
  line L156 (54.0372, 28.1041) -> (54.2641, 28.1041)
  spline S179 degree 2 poles (54.2641, 28.1041) (54.4667, 28.1041) (54.7159, 28.169) (54.7969, 28.2541) knots 0 0 0 1 2 2 2
  spline S180 degree 2 poles (54.7969, 28.2541) (54.8719, 28.329) (54.9388, 28.5053) (54.9388, 28.6248) knots 0 0 0 1 2 2 2
  line L157 (58.0202, 26.8886) -> (56.8006, 26.8886)
  line L158 (56.8006, 26.8886) -> (56.8006, 27.1438)
  line L159 (56.8006, 27.1438) -> (57.2544, 27.1438)
  line L160 (57.2544, 27.1438) -> (57.2544, 28.8193)
  line L161 (57.2544, 28.8193) -> (56.8006, 28.8193)
  line L162 (56.8006, 28.8193) -> (56.8006, 29.0482)
  spline S181 degree 2 poles (56.8006, 29.0482) (57.0579, 29.0482) (57.301, 29.1941) (57.3172, 29.3967) knots 0 0 0 1 2 2 2
  line L163 (57.3172, 29.3967) -> (57.5765, 29.3967)
  line L164 (57.5765, 29.3967) -> (57.5765, 27.1438)
  line L165 (57.5765, 27.1438) -> (58.0202, 27.1438)
  line L166 (58.0202, 27.1438) -> (58.0202, 26.8886)
  line L167 (59.8962, 26.8886) -> (58.6766, 26.8886)
  line L168 (58.6766, 26.8886) -> (58.6766, 27.1438)
  line L169 (58.6766, 27.1438) -> (59.1304, 27.1438)
  line L170 (59.1304, 27.1438) -> (59.1304, 28.8193)
  line L171 (59.1304, 28.8193) -> (58.6766, 28.8193)
  line L172 (58.6766, 28.8193) -> (58.6766, 29.0482)
  spline S182 degree 2 poles (58.6766, 29.0482) (58.9339, 29.0482) (59.177, 29.1941) (59.1932, 29.3967) knots 0 0 0 1 2 2 2
  line L173 (59.1932, 29.3967) -> (59.4525, 29.3967)
  line L174 (59.4525, 29.3967) -> (59.4525, 27.1438)
  line L175 (59.4525, 27.1438) -> (59.8962, 27.1438)
  line L176 (59.8962, 27.1438) -> (59.8962, 26.8886)
  line L177 (60.893, 26.8886) -> (60.4918, 26.8886)
  line L178 (60.4918, 26.8886) -> (60.4918, 27.3667)
  line L179 (60.4918, 27.3667) -> (60.893, 27.3667)
  line L180 (60.893, 27.3667) -> (60.893, 26.8886)
  line L181 (62.8136, 26.8886) -> (61.5939, 26.8886)
  line L182 (61.5939, 26.8886) -> (61.5939, 27.1438)
  line L183 (61.5939, 27.1438) -> (62.0478, 27.1438)
  line L184 (62.0478, 27.1438) -> (62.0478, 28.8193)
  line L185 (62.0478, 28.8193) -> (61.5939, 28.8193)
  line L186 (61.5939, 28.8193) -> (61.5939, 29.0482)
  spline S183 degree 2 poles (61.5939, 29.0482) (61.8512, 29.0482) (62.0943, 29.1941) (62.1106, 29.3967) knots 0 0 0 1 2 2 2
  line L187 (62.1106, 29.3967) -> (62.3699, 29.3967)
  line L188 (62.3699, 29.3967) -> (62.3699, 27.1438)
  line L189 (62.3699, 27.1438) -> (62.8136, 27.1438)
  line L190 (62.8136, 27.1438) -> (62.8136, 26.8886)
  line L191 (65.1576, 29.3886) -> (64.2965, 26.8886)
  line L192 (64.2965, 26.8886) -> (63.9379, 26.8886)
  line L193 (63.9379, 26.8886) -> (63.0769, 29.3886)
  line L194 (63.0769, 29.3886) -> (63.4335, 29.3886)
  line L195 (63.4335, 29.3886) -> (64.1264, 27.312)
  line L196 (64.1264, 27.312) -> (64.8192, 29.3886)
  line L197 (64.8192, 29.3886) -> (65.1576, 29.3886)
  line L198 (67.9412, 26.8886) -> (66.3995, 26.8886)
  line L199 (66.3995, 26.8886) -> (66.3995, 27.2431)
  spline S184 degree 2 poles (66.3995, 27.2431) (66.5656, 27.3991) (66.8614, 27.6888) (67.0032, 27.8448) knots 0 0 0 1 2 2 2
  spline S185 degree 2 poles (67.0032, 27.8448) (67.2888, 28.1588) (67.4975, 28.5357) (67.4975, 28.7362) knots 0 0 0 1 2 2 2
  spline S186 degree 2 poles (67.4975, 28.7362) (67.4975, 28.8416) (67.4327, 28.9996) (67.3739, 29.0502) knots 0 0 0 1 2 2 2
  spline S187 degree 2 poles (67.3739, 29.0502) (67.3152, 29.1009) (67.1612, 29.1515) (67.068, 29.1515) knots 0 0 0 1 2 2 2
  spline S188 degree 2 poles (67.068, 29.1515) (66.9789, 29.1515) (66.7965, 29.107) (66.7135, 29.0725) knots 0 0 0 1 2 2 2
  spline S189 degree 2 poles (66.7135, 29.0725) (66.6426, 29.0442) (66.5109, 28.9631) (66.4704, 28.9348) knots 0 0 0 1 2 2 2
  line L200 (66.4704, 28.9348) -> (66.4521, 28.9348)
  line L201 (66.4521, 28.9348) -> (66.4521, 29.2913)
  spline S190 degree 2 poles (66.4521, 29.2913) (66.5555, 29.342) (66.9262, 29.4412) (67.0923, 29.4412) knots 0 0 0 1 2 2 2
  spline S191 degree 2 poles (67.0923, 29.4412) (67.4428, 29.4412) (67.8379, 29.0705) (67.8379, 28.7545) knots 0 0 0 1 2 2 2
  spline S192 degree 2 poles (67.8379, 28.7545) (67.8379, 28.6066) (67.769, 28.3594) (67.7082, 28.2541) knots 0 0 0 1 2 2 2
  spline S193 degree 2 poles (67.7082, 28.2541) (67.6474, 28.1447) (67.4712, 27.9299) (67.3739, 27.8266) knots 0 0 0 1 2 2 2
  spline S194 degree 2 poles (67.3739, 27.8266) (67.2159, 27.6544) (66.829, 27.2857) (66.7135, 27.1783) knots 0 0 0 1 2 2 2
  line L202 (66.7135, 27.1783) -> (67.9412, 27.1783)
  line L203 (67.9412, 27.1783) -> (67.9412, 26.8886)
  line L204 (69.8456, 29.0138) -> (68.7637, 26.8886)
  line L205 (68.7637, 26.8886) -> (68.4072, 26.8886)
  line L206 (68.4072, 26.8886) -> (69.5498, 29.0948)
  line L207 (69.5498, 29.0948) -> (68.2593, 29.0948)
  line L208 (68.2593, 29.0948) -> (68.2593, 29.3886)
  line L209 (68.2593, 29.3886) -> (69.8456, 29.3886)
  line L210 (69.8456, 29.3886) -> (69.8456, 29.0138)
  spline S195 degree 2 poles (71.7074, 28.1386) (71.7074, 27.466) (71.3164, 26.8359) (70.9092, 26.8359) knots 0 0 0 1 2 2 2
  spline S196 degree 2 poles (70.9092, 26.8359) (70.4959, 26.8359) (70.1089, 27.4781) (70.1089, 28.1365) knots 0 0 0 1 2 2 2
  spline S197 degree 2 poles (70.1089, 28.1365) (70.1089, 28.8132) (70.4999, 29.4392) (70.9092, 29.4392) knots 0 0 0 1 2 2 2
  spline S198 degree 2 poles (70.9092, 29.4392) (71.3204, 29.4392) (71.7074, 28.7909) (71.7074, 28.1386) knots 0 0 0 1 2 2 2
  spline S199 degree 2 poles (71.2779, 27.3768) (71.3265, 27.5004) (71.367, 27.8813) (71.367, 28.1386) knots 0 0 0 1 2 2 2
  spline S200 degree 2 poles (71.367, 28.1386) (71.367, 28.3959) (71.3265, 28.7747) (71.2759, 28.9024) knots 0 0 0 1 2 2 2
  spline S201 degree 2 poles (71.2759, 28.9024) (71.2252, 29.03) (71.049, 29.1617) (70.9092, 29.1617) knots 0 0 0 1 2 2 2
  spline S202 degree 2 poles (70.9092, 29.1617) (70.7694, 29.1617) (70.5891, 29.03) (70.5364, 28.8983) knots 0 0 0 1 2 2 2
  spline S203 degree 2 poles (70.5364, 28.8983) (70.4858, 28.7707) (70.4493, 28.3817) (70.4493, 28.1365) knots 0 0 0 1 2 2 2
  spline S204 degree 2 poles (70.4493, 28.1365) (70.4493, 27.8732) (70.4817, 27.5207) (70.5344, 27.3829) knots 0 0 0 1 2 2 2
  spline S205 degree 2 poles (70.5344, 27.3829) (70.583, 27.2532) (70.7633, 27.1135) (70.9092, 27.1135) knots 0 0 0 1 2 2 2
  spline S206 degree 2 poles (70.9092, 27.1135) (71.0469, 27.1135) (71.2273, 27.2451) (71.2779, 27.3768) knots 0 0 0 1 2 2 2
  spline S207 degree 2 poles (73.5834, 28.1386) (73.5834, 27.466) (73.1924, 26.8359) (72.7852, 26.8359) knots 0 0 0 1 2 2 2
  spline S208 degree 2 poles (72.7852, 26.8359) (72.3719, 26.8359) (71.9849, 27.4781) (71.9849, 28.1365) knots 0 0 0 1 2 2 2
  spline S209 degree 2 poles (71.9849, 28.1365) (71.9849, 28.8132) (72.376, 29.4392) (72.7852, 29.4392) knots 0 0 0 1 2 2 2
  spline S210 degree 2 poles (72.7852, 29.4392) (73.1965, 29.4392) (73.5834, 28.7909) (73.5834, 28.1386) knots 0 0 0 1 2 2 2
  spline S211 degree 2 poles (73.1539, 27.3768) (73.2025, 27.5004) (73.2431, 27.8813) (73.2431, 28.1386) knots 0 0 0 1 2 2 2
  spline S212 degree 2 poles (73.2431, 28.1386) (73.2431, 28.3959) (73.2025, 28.7747) (73.1519, 28.9024) knots 0 0 0 1 2 2 2
  spline S213 degree 2 poles (73.1519, 28.9024) (73.1012, 29.03) (72.925, 29.1617) (72.7852, 29.1617) knots 0 0 0 1 2 2 2
  spline S214 degree 2 poles (72.7852, 29.1617) (72.6454, 29.1617) (72.4651, 29.03) (72.4124, 28.8983) knots 0 0 0 1 2 2 2
  spline S215 degree 2 poles (72.4124, 28.8983) (72.3618, 28.7707) (72.3253, 28.3817) (72.3253, 28.1365) knots 0 0 0 1 2 2 2
  spline S216 degree 2 poles (72.3253, 28.1365) (72.3253, 27.8732) (72.3577, 27.5207) (72.4104, 27.3829) knots 0 0 0 1 2 2 2
  spline S217 degree 2 poles (72.4104, 27.3829) (72.459, 27.2532) (72.6393, 27.1135) (72.7852, 27.1135) knots 0 0 0 1 2 2 2
  spline S218 degree 2 poles (72.7852, 27.1135) (72.923, 27.1135) (73.1033, 27.2451) (73.1539, 27.3768) knots 0 0 0 1 2 2 2
  line L211 (76.0773, 26.8886) -> (76.0773, 27.9745)
  spline S219 degree 2 poles (76.0773, 27.9745) (76.0773, 28.1041) (76.0571, 28.325) (76.0247, 28.3857) knots 0 0 0 1 2 2 2
  spline S220 degree 2 poles (76.0247, 28.3857) (75.9922, 28.4526) (75.8687, 28.5174) (75.7613, 28.5174) knots 0 0 0 1 2 2 2
  spline S221 degree 2 poles (75.7613, 28.5174) (75.664, 28.5174) (75.4412, 28.3979) (75.3237, 28.2844) knots 0 0 0 1 2 2 2
  spline S222 degree 2 poles (75.3237, 28.2844) (75.3257, 28.2561) (75.3298, 28.1771) (75.3298, 28.1244) knots 0 0 0 1 2 2 2
  line L212 (75.3298, 28.1244) -> (75.3298, 26.8886)
  line L213 (75.3298, 26.8886) -> (75.0137, 26.8886)
  line L214 (75.0137, 26.8886) -> (75.0137, 27.9745)
  spline S223 degree 2 poles (75.0137, 27.9745) (75.0137, 28.1041) (74.9935, 28.325) (74.961, 28.3857) knots 0 0 0 1 2 2 2
  spline S224 degree 2 poles (74.961, 28.3857) (74.9286, 28.4526) (74.805, 28.5174) (74.6977, 28.5174) knots 0 0 0 1 2 2 2
  spline S225 degree 2 poles (74.6977, 28.5174) (74.5964, 28.5174) (74.3715, 28.3898) (74.2661, 28.2905) knots 0 0 0 1 2 2 2
  line L215 (74.2661, 28.2905) -> (74.2661, 26.8886)
  line L216 (74.2661, 26.8886) -> (73.9501, 26.8886)
  line L217 (73.9501, 26.8886) -> (73.9501, 28.7646)
  line L218 (73.9501, 28.7646) -> (74.2661, 28.7646)
  line L219 (74.2661, 28.7646) -> (74.2661, 28.5579)
  spline S226 degree 2 poles (74.2661, 28.5579) (74.3897, 28.6815) (74.6328, 28.8173) (74.7787, 28.8173) knots 0 0 0 1 2 2 2
  spline S227 degree 2 poles (74.7787, 28.8173) (74.9448, 28.8173) (75.2021, 28.6653) (75.269, 28.4931) knots 0 0 0 1 2 2 2
  spline S228 degree 2 poles (75.269, 28.4931) (75.4128, 28.6532) (75.6843, 28.8173) (75.8423, 28.8173) knots 0 0 0 1 2 2 2
  spline S229 degree 2 poles (75.8423, 28.8173) (75.9639, 28.8173) (76.1624, 28.7423) (76.2354, 28.6572) knots 0 0 0 1 2 2 2
  spline S230 degree 2 poles (76.2354, 28.6572) (76.3103, 28.5721) (76.3934, 28.3169) (76.3934, 28.1244) knots 0 0 0 1 2 2 2
  line L220 (76.3934, 28.1244) -> (76.3934, 26.8886)
  line L221 (76.3934, 26.8886) -> (76.0773, 26.8886)
  line L222 (76.5919, 26.8886) -> (77.4347, 29.3886)
  line L223 (77.4347, 29.3886) -> (77.8439, 29.3886)
  line L224 (77.8439, 29.3886) -> (78.6867, 26.8886)
  line L225 (78.6867, 26.8886) -> (78.3362, 26.8886)
  line L226 (78.3362, 26.8886) -> (78.1093, 27.5875)
  line L227 (78.1093, 27.5875) -> (77.1551, 27.5875)
  line L228 (77.1551, 27.5875) -> (76.9282, 26.8886)
  line L229 (76.9282, 26.8886) -> (76.5919, 26.8886)
  line L230 (78.0182, 27.8712) -> (77.6312, 29.0482)
  line L231 (77.6312, 29.0482) -> (77.2463, 27.8712)
  line L232 (77.2463, 27.8712) -> (78.0182, 27.8712)
  line L233 (80.3723, 26.8886) -> (80.0563, 26.8886)
  line L234 (80.0563, 26.8886) -> (80.0563, 27.9583)
  spline S231 degree 2 poles (80.0563, 27.9583) (80.0563, 28.0879) (80.032, 28.3108) (79.9955, 28.3776) knots 0 0 0 1 2 2 2
  spline S232 degree 2 poles (79.9955, 28.3776) (79.957, 28.4485) (79.8192, 28.5174) (79.7017, 28.5174) knots 0 0 0 1 2 2 2
  spline S233 degree 2 poles (79.7017, 28.5174) (79.5842, 28.5174) (79.335, 28.3918) (79.2155, 28.2905) knots 0 0 0 1 2 2 2
  line L235 (79.2155, 28.2905) -> (79.2155, 26.8886)
  line L236 (79.2155, 26.8886) -> (78.8995, 26.8886)
  line L237 (78.8995, 26.8886) -> (78.8995, 29.5)
  line L238 (78.8995, 29.5) -> (79.2155, 29.5)
  line L239 (79.2155, 29.5) -> (79.2155, 28.5559)
  spline S234 degree 2 poles (79.2155, 28.5559) (79.3573, 28.6835) (79.6308, 28.8173) (79.7848, 28.8173) knots 0 0 0 1 2 2 2
  spline S235 degree 2 poles (79.7848, 28.8173) (80.0603, 28.8173) (80.3723, 28.4526) (80.3723, 28.1062) knots 0 0 0 1 2 2 2
  line L240 (80.3723, 28.1062) -> (80.3723, 26.8886)
  line L241 (83.3849, 26.8886) -> (81.8431, 26.8886)
  line L242 (81.8431, 26.8886) -> (81.8431, 27.2431)
  spline S236 degree 2 poles (81.8431, 27.2431) (82.0093, 27.3991) (82.305, 27.6888) (82.4469, 27.8448) knots 0 0 0 1 2 2 2
  spline S237 degree 2 poles (82.4469, 27.8448) (82.7325, 28.1588) (82.9412, 28.5357) (82.9412, 28.7362) knots 0 0 0 1 2 2 2
  spline S238 degree 2 poles (82.9412, 28.7362) (82.9412, 28.8416) (82.8764, 28.9996) (82.8176, 29.0502) knots 0 0 0 1 2 2 2
  spline S239 degree 2 poles (82.8176, 29.0502) (82.7589, 29.1009) (82.6049, 29.1515) (82.5117, 29.1515) knots 0 0 0 1 2 2 2
  spline S240 degree 2 poles (82.5117, 29.1515) (82.4226, 29.1515) (82.2402, 29.107) (82.1572, 29.0725) knots 0 0 0 1 2 2 2
  spline S241 degree 2 poles (82.1572, 29.0725) (82.0862, 29.0442) (81.9546, 28.9631) (81.914, 28.9348) knots 0 0 0 1 2 2 2
  line L243 (81.914, 28.9348) -> (81.8958, 28.9348)
  line L244 (81.8958, 28.9348) -> (81.8958, 29.2913)
  spline S242 degree 2 poles (81.8958, 29.2913) (81.9991, 29.342) (82.3699, 29.4412) (82.536, 29.4412) knots 0 0 0 1 2 2 2
  spline S243 degree 2 poles (82.536, 29.4412) (82.8865, 29.4412) (83.2815, 29.0705) (83.2815, 28.7545) knots 0 0 0 1 2 2 2
  spline S244 degree 2 poles (83.2815, 28.7545) (83.2815, 28.6066) (83.2127, 28.3594) (83.1519, 28.2541) knots 0 0 0 1 2 2 2
  spline S245 degree 2 poles (83.1519, 28.2541) (83.0911, 28.1447) (82.9149, 27.9299) (82.8176, 27.8266) knots 0 0 0 1 2 2 2
  spline S246 degree 2 poles (82.8176, 27.8266) (82.6596, 27.6544) (82.2726, 27.2857) (82.1572, 27.1783) knots 0 0 0 1 2 2 2
  line L245 (82.1572, 27.1783) -> (83.3849, 27.1783)
  line L246 (83.3849, 27.1783) -> (83.3849, 26.8886)
  spline S247 degree 2 poles (83.6503, 28.5762) (83.6503, 28.7686) (83.7759, 29.0887) (83.8853, 29.2042) knots 0 0 0 1 2 2 2
  spline S248 degree 2 poles (83.8853, 29.2042) (83.9886, 29.3156) (84.2905, 29.4392) (84.4444, 29.4392) knots 0 0 0 1 2 2 2
  spline S249 degree 2 poles (84.4444, 29.4392) (84.6166, 29.4392) (84.8962, 29.3237) (84.9995, 29.2143) knots 0 0 0 1 2 2 2
  spline S250 degree 2 poles (84.9995, 29.2143) (85.1292, 29.0766) (85.271, 28.6309) (85.271, 28.2885) knots 0 0 0 1 2 2 2
  spline S251 degree 2 poles (85.271, 28.2885) (85.271, 27.9785) (85.1312, 27.4234) (84.9955, 27.2391) knots 0 0 0 1 2 2 2
  spline S252 degree 2 poles (84.9955, 27.2391) (84.8516, 27.0446) (84.4465, 26.84) (84.1507, 26.84) knots 0 0 0 1 2 2 2
  spline S253 degree 2 poles (84.1507, 26.84) (84.0838, 26.84) (83.9319, 26.8541) (83.867, 26.8744) knots 0 0 0 1 2 2 2
  line L247 (83.867, 26.8744) -> (83.867, 27.1965)
  line L248 (83.867, 27.1965) -> (83.8832, 27.1965)
  spline S254 degree 2 poles (83.8832, 27.1965) (83.9258, 27.1722) (84.1041, 27.1297) (84.1952, 27.1297) knots 0 0 0 1 2 2 2
  spline S255 degree 2 poles (84.1952, 27.1297) (84.5234, 27.1297) (84.8982, 27.5632) (84.9246, 27.9643) knots 0 0 0 1 2 2 2
  spline S256 degree 2 poles (84.9246, 27.9643) (84.7909, 27.8732) (84.5478, 27.7901) (84.4039, 27.7901) knots 0 0 0 1 2 2 2
  spline S257 degree 2 poles (84.4039, 27.7901) (84.2661, 27.7901) (84.0372, 27.8509) (83.9217, 27.938) knots 0 0 0 1 2 2 2
  spline S258 degree 2 poles (83.9217, 27.938) (83.788, 28.0413) (83.6503, 28.3553) (83.6503, 28.5762) knots 0 0 0 1 2 2 2
  spline S259 degree 2 poles (84.9327, 28.3635) (84.9327, 28.6167) (84.8395, 28.9368) (84.7564, 29.0239) knots 0 0 0 1 2 2 2
  spline S260 degree 2 poles (84.7564, 29.0239) (84.6835, 29.1049) (84.5315, 29.1657) (84.4424, 29.1657) knots 0 0 0 1 2 2 2
  spline S261 degree 2 poles (84.4424, 29.1657) (84.2358, 29.1657) (83.9906, 28.8699) (83.9906, 28.5904) knots 0 0 0 1 2 2 2
  spline S262 degree 2 poles (83.9906, 28.5904) (83.9906, 28.4323) (84.0717, 28.2277) (84.1608, 28.1548) knots 0 0 0 1 2 2 2
  spline S263 degree 2 poles (84.1608, 28.1548) (84.2256, 28.1021) (84.3857, 28.0677) (84.4789, 28.0677) knots 0 0 0 1 2 2 2
  spline S264 degree 2 poles (84.4789, 28.0677) (84.5862, 28.0677) (84.8334, 28.1426) (84.9266, 28.2054) knots 0 0 0 1 2 2 2
  spline S265 degree 2 poles (84.9266, 28.2054) (84.9286, 28.2297) (84.9327, 28.3128) (84.9327, 28.3635) knots 0 0 0 1 2 2 2
  line L249 (86.132, 26.8886) -> (85.7309, 26.8886)
  line L250 (85.7309, 26.8886) -> (85.7309, 27.3667)
  line L251 (85.7309, 27.3667) -> (86.132, 27.3667)
  line L252 (86.132, 27.3667) -> (86.132, 26.8886)
  spline S266 degree 2 poles (86.5676, 28.5762) (86.5676, 28.7686) (86.6932, 29.0887) (86.8026, 29.2042) knots 0 0 0 1 2 2 2
  spline S267 degree 2 poles (86.8026, 29.2042) (86.9059, 29.3156) (87.2078, 29.4392) (87.3618, 29.4392) knots 0 0 0 1 2 2 2
  spline S268 degree 2 poles (87.3618, 29.4392) (87.534, 29.4392) (87.8136, 29.3237) (87.9169, 29.2143) knots 0 0 0 1 2 2 2
  spline S269 degree 2 poles (87.9169, 29.2143) (88.0465, 29.0766) (88.1884, 28.6309) (88.1884, 28.2885) knots 0 0 0 1 2 2 2
  spline S270 degree 2 poles (88.1884, 28.2885) (88.1884, 27.9785) (88.0486, 27.4234) (87.9128, 27.2391) knots 0 0 0 1 2 2 2
  spline S271 degree 2 poles (87.9128, 27.2391) (87.769, 27.0446) (87.3638, 26.84) (87.068, 26.84) knots 0 0 0 1 2 2 2
  spline S272 degree 2 poles (87.068, 26.84) (87.0012, 26.84) (86.8492, 26.8541) (86.7844, 26.8744) knots 0 0 0 1 2 2 2
  line L253 (86.7844, 26.8744) -> (86.7844, 27.1965)
  line L254 (86.7844, 27.1965) -> (86.8006, 27.1965)
  spline S273 degree 2 poles (86.8006, 27.1965) (86.8431, 27.1722) (87.0214, 27.1297) (87.1126, 27.1297) knots 0 0 0 1 2 2 2
  spline S274 degree 2 poles (87.1126, 27.1297) (87.4408, 27.1297) (87.8156, 27.5632) (87.8419, 27.9643) knots 0 0 0 1 2 2 2
  spline S275 degree 2 poles (87.8419, 27.9643) (87.7082, 27.8732) (87.4651, 27.7901) (87.3213, 27.7901) knots 0 0 0 1 2 2 2
  spline S276 degree 2 poles (87.3213, 27.7901) (87.1835, 27.7901) (86.9546, 27.8509) (86.8391, 27.938) knots 0 0 0 1 2 2 2
  spline S277 degree 2 poles (86.8391, 27.938) (86.7054, 28.0413) (86.5676, 28.3553) (86.5676, 28.5762) knots 0 0 0 1 2 2 2